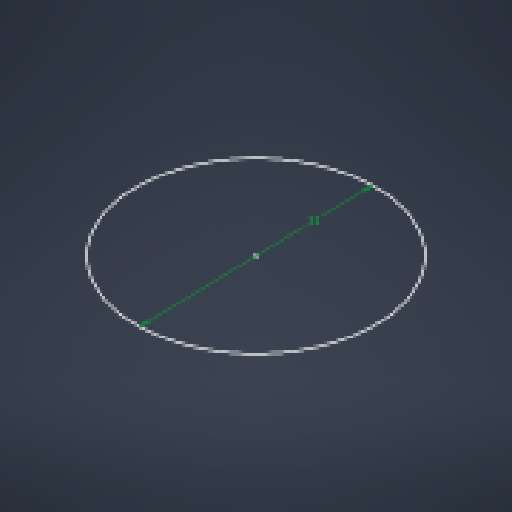
# Autodesk Inventor part: Battery Cover
Saved by Autodesk Inventor 2026.1 (Build 301233020, 233B)
## iProperties
Created: 2025-09-16
Part Number: Battery Cover
Material: Generic
Document SubType Name: Modeling
Designer: Administrator
Density: 1 g/cm^3
Appearance: Default
Author: Administrator
Autodesk Inventor part; units mm, degrees
ref_plane "YZ Plane" through (0, 0, 0) normal (1, 0, 0) x (0, 1, 0)
ref_plane "XZ Plane" through (0, 0, 0) normal (0, 1, 0) x (-1, 0, 0)
ref_plane "XY Plane" through (0, 0, 0) normal (0, 0, 1) x (1, 0, 0)
sketch "Sketch1" plane through (0, 0, 0) normal (0, 1, 0) x (-1, 0, 0)
  circle A0 centre (0, 0) radius 32
  line L0 (27.5, 0) -> (-27.5, 0) construction
  circle A1 centre (27.5, 0) radius 3.5
  circle A2 centre (-27.5, 0) radius 3.5
  line L1 (26, 32) -> (-26, 32)
  line L2 (-26, 32) -> (-26, -32)
  line L3 (-26, -32) -> (26, -32)
  line L4 (26, -32) -> (26, 32)
  line L5 (26, 32) -> (-26, -32) construction
  line L6 (-26, 32) -> (26, -32) construction
  line L7 (0, -32) -> (0, -13) construction
  line L8 (7.5, -32) -> (7.5, -13)
  line L9 (-7.5, -13) -> (-7.5, -32)
  arc A3 (-7.5, -32) -> (7.5, -32) centre (0, -32) ccw
  arc A4 (7.5, -13) -> (-7.5, -13) centre (0, -13) ccw
  line L10 (-28.2666, 32) -> (28.2666, 32)
  line L11 (28.2666, 32) -> (28.2666, 15)
  line L12 (28.2666, 15) -> (-28.2666, 15)
  line L13 (-28.2666, 15) -> (-28.2666, 32)
  point P0 (0, -22.5)
  point P1 (0, -5.5)
  point P2 (31, 0)
  point P3 (-31, 0)
  point P4 (-7.5, -31.1087)
  point P5 (7.5, -31.1087)
  dimension "d0" = 64
  dimension "d1" = 55
  dimension "d2" = 7
  dimension "d3" = 7
  dimension "d4" = 52
  dimension "d5" = 15
  dimension "d6" = 5.5
  dimension "d13" = 15
  constraints: 30 end point, 7 point on circle, 6 coincident, 5 centre point, 5 midpoint, 5 parallel, 5 tangent, 3 horizontal, 3 perpendicular, 1 point on line
  measures "d0" diameter of A0
  measures "d1" distance of L0.start L0.end
  measures "d2" diameter of A1
  measures "d3" diameter of A2
  measures "d4" distance of L3.end L2.end
  measures "d5" diameter of A4
  measures "d6" distance from line of L0 point (0, -5.5)
  measures "d13" distance between parallel lines of L0 L12
extrude "Extrusion1" add sketch "Sketch1" along normal blind 1 contours A0 L4 A1 L12 | A0 L8 A4 L9 L2 A2 L12 L4 A1 | L2 A2 A0 L12
fillet "Fillet1" radius 1 4 edges at (-7.5, 0.5, -31.1087) (7.5, 0.5, -31.1087) (-28.2666, 0.5, 15) (28.2666, 0.5, 15)
chamfer "Chamfer1" distance 0.25 angle 45 20 edges at (-24, 0, 0) (-24, 1, 0) (29.3193, 1, -12.8211) (7.8976, 1, -30.6101) (7.5, 1, -21.406) (0, 1, -5.5) (-7.5, 1, -21.406) (-7.8976, 1, -30.6101) (-29.3193, 1, -12.8211) (-29.3193, 0, -12.8211) (-7.8976, 0, -30.6101) (-7.5, 0, -21.406) (0, 0, -5.5) (7.5, 0, -21.406) (7.8976, 0, -30.6101) (29.3193, 0, -12.8211) (31, 0, 0) (31, 1, 0) (0, 0, 15) (0, 1, 15)
body "Solid1"
